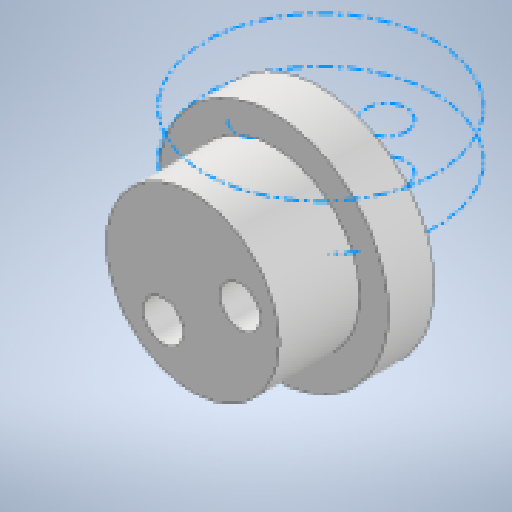
# Autodesk Inventor part: Shaft-2
Saved by Autodesk Inventor 2023 (Build 270158000, 158)
## iProperties
Created: 2023-01-17
Part Number: Shaft-2
Material: Generic
Document SubType Name: Modeling
Designer: caden
Density: 1 g/cm^3
Appearance: Default
Author: caden
Autodesk Inventor part; units mm, degrees
ref_plane "YZ Plane" through (0, 0, 0) normal (1, 0, 0) x (0, 1, 0)
ref_plane "XZ Plane" through (0, 0, 0) normal (0, 1, 0) x (-1, 0, 0)
ref_plane "XY Plane" through (0, 0, 0) normal (0, 0, 1) x (1, 0, 0)
sketch "Sketch3" plane through (0, 0, 0) normal (0, 0, 1) x (1, 0, 0)
  circle A0 centre (-0.1954, 1.4872) radius 10
  circle A1 centre (0.5933, 0.2945) radius 7.5 construction
  circle A2 centre (-2.7432, -1.9118) radius 1.75 construction
  circle A3 centre (-2.7432, -1.9118) radius 1.75
  circle A4 centre (3.9298, 2.5008) radius 1.75
  circle A5 centre (3.9298, 2.5008) radius 1.75 construction
  line L0 (3.9298, 2.5008) -> (-2.7432, -1.9118) construction
  line L1 (0.5933, 0.2945) -> (-1.1822, 2.9794) construction
  point P0 (0, 0)
  dimension "d1" = 1.5
  dimension "d2" = 20
  dimension "d9" = 8
  constraints: 4 end point, 3 centre point, 2 coincident, 2 equal radius, 1 perpendicular, 1 point on line
  measures "d1" distance of A0.centre point (0, 0)
  measures "d2" diameter of A0
  measures "d9" distance of L0.start L0.end
extrude "Extrusion1" add sketch "Sketch3" along normal blind 4
sketch "Sketch4" plane through (-0.1954, 1.4872, 4) normal (0, 0, 1) x (1, 0, 0)
  circle A0 centre (0, 0) radius 10 construction
  circle A1 centre (4.1252, 1.0136) radius 1.75 construction
  circle A2 centre (-2.5478, -3.399) radius 1.75 construction
  circle A3 centre (0, 0) radius 7.5
  circle A4 centre (4.1252, 1.0136) radius 1.75
  circle A5 centre (-2.5478, -3.399) radius 1.75
  point P0 (0.1954, -1.4872)
  dimension "d6" = 15
  constraints: 3 centre point, 3 coincident, 1 concentric
  measures "d6" diameter of A3
extrude "Extrusion2" add sketch "Sketch4" along normal blind 7
body "Solid1"
